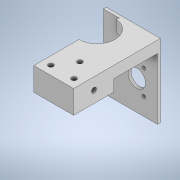
# Autodesk Inventor part: motor_connector_left
Saved by Autodesk Inventor 2021 (Build 250183000, 183)
## iProperties
Created: 2020-11-22
Part Number: motor_connector_left
Material: Generic
Document SubType Name: Modeling
Designer: Mateusz
Density: 1 g/cm^3
Appearance: Default
Author: Mateusz
Autodesk Inventor part; units mm, degrees
ref_plane "YZ Plane" through (0, 0, 0) normal (1, 0, 0) x (0, 1, 0)
ref_plane "XZ Plane" through (0, 0, 0) normal (0, 1, 0) x (-1, 0, 0)
ref_plane "Work Plane1" through (8.5, -35.5, -35.5) normal (0, 0, -1) x (-1, 0, 0)
sketch "Sketch1" plane through (8.5, -35.5, -35.5) normal (0, 0, -1) x (-1, 0, 0)
  circle A0 centre (0, 0) radius 3 projected
  circle A1 centre (0, 0) radius 6 projected
  circle A2 centre (-36.75, -21.2176) radius 3 projected
  circle A3 centre (-36.75, -21.2176) radius 6 projected
  circle A4 centre (-36.75, 21.2176) radius 6 projected
  circle A5 centre (-36.75, 21.2176) radius 3 projected
  line L0 (-36.75, -46.2176) -> (28, -46.2176)
  line L1 (28, -46.2176) -> (28, 0)
  line L2 (-36.75, -46.2176) -> (-59, -46.2176)
  line L3 (-59, -46.2176) -> (-59, 34.5)
  line L4 (-59, 34.5) -> (28, 34.5)
  line L5 (34.5, 35.5) -> (-17.5, 35.5) projected
  line L6 (28, 34.5) -> (28, 0)
  circle A6 centre (-24.5, 0) radius 11 projected
  circle A7 centre (-24.5, 0) radius 15
  point P0 (8.5, 35.5)
  dimension "d3" = 30
  constraints: 12 end point, 3 perpendicular, 1 centre point, 1 coincident, 1 horizontal, 1 parallel
  measures "d3" diameter of A7
extrude "Extrusion1" add sketch "Sketch1" along normal blind 5 contours A1 | A3 | A4 | L2 L3 L4 L6 L1 L0
sketch "Sketch2" plane through (-19.5, -81.7176, -35.5) normal (-1, 0, 0) x (0, 0, 1)
  line L0 (0, 0) -> (0, 80.7176) projected
  line L1 (0, 80.7176) -> (-5, 80.7176) projected
  line L2 (-5, 0) -> (-5, 80.7176) projected
  line L3 (0, 0) -> (-5, 0) projected
  point P0 (35.5, 81.7176)
extrude "Extrusion2" add sketch "Sketch2" along normal blind 5
sketch "Sketch3" plane through (67.5, -81.7176, -40.5) normal (0, -1, 0) x (1, 0, 0)
  line L0 (0, 5) -> (-92, 5) projected
  line L1 (-92, 0) -> (-92, 5) projected
  line L2 (0, 0) -> (-92, 0) projected
  line L3 (0, 5) -> (0, 0) projected
  point P0 (-67.5, 40.5)
extrude "Extrusion3" add sketch "Sketch3" along normal blind 5
sketch "Sketch4" plane through (8.5, -35.5, -35.5) normal (0, 0, 1) x (1, 0, 0)
  line L0 (-28, -46.2176) -> (-28, 34.5)
  line L1 (-28, -46.2176) -> (59, -46.2176)
  line L2 (59, -51.2176) -> (-33, -51.2176) projected
  line L3 (-33, 34.5) -> (-33, -51.2176) projected
  line L4 (59, 34.5) -> (59, -51.2176) projected
  line L5 (59, 34.5) -> (-33, 34.5) projected
  line L6 (-28, -46.2176) -> (-33, -46.2176)
  line L7 (-33, 34.5) -> (-33, -51.2176) projected
  constraints: 6 end point, 1 perpendicular, 1 point on line
extrude "Extrusion4" add sketch "Sketch4" along normal blind 75 contours L1 L4 L2 L3 L6
sketch "Sketch5" plane through (67.5, -86.7176, -40.5) normal (0, -1, 0) x (1, 0, 0)
  line L0 (-92, 5) -> (-92, 80) projected
  line L1 (-92, 80) -> (-77.75, 80)
  line L2 (-92, 80) -> (0, 80) projected
  line L3 (-77.75, 80) -> (-37.75, 80)
  line L4 (-37.75, 80) -> (-37.75, 65)
  line L5 (-37.75, 65) -> (-77.75, 65)
  circle A0 centre (-77.75, 65) radius 4.25
  circle A1 centre (-37.75, 65) radius 4.25
  point P0 (-67.5, 40.5)
  dimension "d14" = 14.25
  dimension "d15" = 40
  dimension "d16" = 15
  dimension "d17" = 8.5
  dimension "d18" = 8.5
  constraints: 8 end point, 2 centre point, 2 coincident, 2 perpendicular, 2 point on line
  measures "d14" distance of L0.end L1.end
  measures "d15" distance of L1.end L3.end
  measures "d16" distance of L3.end L4.end
  measures "d17" diameter of A0
  measures "d18" diameter of A1
extrude "Extrusion5" cut sketch "Sketch5" against normal through all
sketch "Sketch6" plane through (67.5, -1, -35.5) normal (0, 1, 0) x (1, 0, 0)
  line L0 (0, 0) -> (-92, 0) projected
  line L1 (0, 0) -> (0, 5) projected
  line L2 (0, 5) -> (-92, 5) projected
  line L3 (-92, 0) -> (-92, 5) projected
  point P0 (-67.5, -35.5)
extrude "Extrusion6" add sketch "Sketch6" along normal blind 20
sketch "Sketch7" plane through (67.5, 19, -35.5) normal (0, 1, 0) x (1, 0, 0)
  circle A0 centre (-67.5, -35.5) radius 31 projected
  circle A1 centre (-67.5, -35.5) radius 31 projected
  circle A2 centre (-67.5, -35.5) radius 31 projected
  line L0 (-67.5, -66.5) -> (-67.5, -75)
  line L1 (0, -75) -> (-92, -75) projected
  line L2 (0, 5) -> (0, -75) projected
  line L3 (-67.5, -75) -> (0, -75)
  line L4 (0, -75) -> (0, 5)
  line L5 (-65, -20.5) -> (-65, 0) projected
  line L6 (-65, -4.601) -> (-65, 0)
  line L7 (-92, 5) -> (-92, 0) projected
  line L8 (-92, 0) -> (0, 0) projected
  line L9 (0, 0) -> (0, 5) projected
  line L10 (0, 5) -> (-92, 5) projected
  point P0 (-65, -4.601)
  constraints: 8 end point, 3 point on line, 2 point on circle, 1 collinear, 1 horizontal, 1 vertical
extrude "Extrusion7" add sketch "Sketch7" along normal blind 20 contours A0 L5 L8 L2 L1 L0 | L8 L7 L10 L2
sketch "Sketch10" plane through (8.5, -35.5, 39.5) normal (0, 0, 1) x (1, 0, 0)
  line L0 (59, -51.2176) -> (59, -46.2176) projected
  line L1 (59, -46.2176) -> (-33, -46.2176) projected
  line L2 (-33, -46.2176) -> (-33, -51.2176) projected
  line L3 (-33, -51.2176) -> (59, -51.2176) projected
  point P0 (-8.5, 35.5)
extrude "Extrusion10" cut sketch "Sketch10" against normal up to surface (75 mm away)
sketch "Sketch11" plane through (0, 19, 39.5) normal (0, 0, 1) x (1, 0, 0)
  line L0 (0, 0) -> (67.5, 0) projected
  line L1 (67.5, 0) -> (67.5, 20) projected
  line L2 (0, 20) -> (67.5, 20) projected
  line L3 (0, 0) -> (0, 20) projected
  point P0 (0, -19)
extrude "Extrusion11" add sketch "Sketch11" along normal blind 10
sketch "Sketch12" plane through (67.5, 19, -35.5) normal (0, -1, 0) x (1, 0, 0)
  line L0 (-67.5, 66.5) -> (-67.5, 85) projected
  line L1 (-67.5, 85) -> (0, 85) projected
  line L2 (-67.5, 85) -> (0, 85)
  line L3 (0, 85) -> (0, 75)
  line L4 (0, 0) -> (0, 85) projected
  line L5 (0, 75) -> (-67.5, 75)
  line L6 (-67.5, 75) -> (-67.5, 85)
  point P0 (-67.5, 35.5)
  dimension "d35" = 10
  constraints: 8 end point, 2 perpendicular, 1 horizontal, 1 point on line
  measures "d35" distance of L1.end L3.end
extrude "Extrusion12" add sketch "Sketch12" along normal blind 20
sketch "Sketch13" plane through (0, 19, 49.5) normal (0, 0, 1) x (1, 0, 0)
  line L0 (67.5, 20) -> (67.5, -20) projected
  line L1 (67.5, 20) -> (0, 20) projected
  line L2 (0, 20) -> (0, -20) projected
  line L3 (67.5, -20) -> (0, -20) projected
  point P0 (0, -19)
extrude "Extrusion13" add sketch "Sketch13" along normal blind 59.488
sketch "Sketch14" plane through (67.5, -1, -35.5) normal (0, -1, 0) x (1, 0, 0)
  line L0 (-53.25, 129.488) -> (-13.25, 129.488)
  circle A0 centre (-53.25, 129.488) radius 4.25
  circle A1 centre (-13.25, 129.488) radius 4.25
  point P0 (-67.5, 35.5)
  point P1 (-67.5, 144.488)
  dimension "d43" = 40
  dimension "d44" = 8.5
  dimension "d45" = 8.5
  constraints: 2 centre point, 2 coincident, 2 end point
  measures "d43" distance of L0.start L0.end
  measures "d44" diameter of A0
  measures "d45" diameter of A1
extrude "Extrusion14" cut sketch "Sketch14" against normal up to surface (40 mm away)
sketch "Sketch15" plane through (67.5, -86.7176, -40.5) normal (1, 0, 0) x (0, 0, -1)
  line L0 (-5, 105.7176) -> (-5, 0) projected
  line L1 (0, 0) -> (-5, 0) projected
  line L2 (0, 0) -> (0, 125.7176) projected
  line L3 (0, 125.7176) -> (-149.488, 125.7176) projected
  line L4 (-149.488, 85.7176) -> (-149.488, 125.7176) projected
  line L5 (-80, 85.7176) -> (-149.488, 85.7176) projected
  line L6 (-80, 105.7176) -> (-80, 85.7176) projected
  line L7 (-5, 105.7176) -> (-80, 105.7176) projected
  point P0 (-40.5, 86.7176)
extrude "Extrusion15" add sketch "Sketch15" along normal blind 1
sketch "Sketch16" plane through (0, 19, 31) normal (-1, 0, 0) x (0, 0, 1)
  line L0 (77.988, 20) -> (77.988, -20) projected
  line L1 (77.988, 0) -> (42.988, 0)
  circle A0 centre (42.988, 0) radius 4.25
  point P0 (-31, -19)
  dimension "d50" = 35
  dimension "d51" = 8.5
  constraints: 2 end point, 1 centre point, 1 coincident, 1 horizontal, 1 midpoint
  measures "d50" distance of L1.start L1.end
  measures "d51" diameter of A0
extrude "Extrusion16" cut sketch "Sketch16" against normal up to surface (68.5 mm away)
sketch "Sketch17" plane through (67.5, 39, -35.5) normal (0, 1, 0) x (1, 0, 0)
  circle A0 centre (-53.25, -129.488) radius 4.25 projected
  line L0 (-53.25, -129.488) -> (-33.25, -129.488)
  line L1 (-33.25, -129.488) -> (-33.25, -99.488)
  circle A1 centre (-33.25, -99.488) radius 4.25
  point P0 (-67.5, -35.5)
  dimension "d54" = 20
  dimension "d55" = 30
  dimension "d56" = 8.5
  constraints: 4 end point, 1 centre point, 1 coincident, 1 horizontal, 1 vertical
  measures "d54" distance of L0.start L0.end
  measures "d55" distance of L0.end L1.end
  measures "d56" diameter of A1
extrude "Extrusion17" cut sketch "Sketch17" against normal up to surface (40 mm away) contours A1
body "Solid1"
